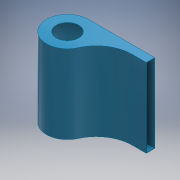
# Autodesk Inventor part: blower
Saved by Autodesk Inventor 2017 (Build 210142000, 142)
## iProperties
Created: 2017-04-22
Part Number: blower
Material: Generic
Document SubType Name: Modeling
Designer: master
Density: 1 g/cm^3
Appearance: Sky Blue Dark
Author: master
Autodesk Inventor part; units mm, degrees
ref_plane "YZ Plane" through (0, 0, 0) normal (1, 0, 0) x (0, 1, 0)
ref_plane "XZ Plane" through (0, 0, 0) normal (0, 1, 0) x (-1, 0, 0)
ref_plane "XY Plane" through (0, 0, 0) normal (0, 0, 1) x (1, 0, 0)
sketch "Sketch1" plane through (0, 0, 0) normal (0, 0, 1) x (1, 0, 0)
  arc A0 (0, 7.5) -> (6.8483, -3.0578) centre (0, 0) ccw
  line L0 (0, 7.5) -> (23.5, 7.5)
  line L1 (23.5, 7.5) -> (23.5, 4.5)
  line L2 (23.5, 4.5) -> (18.5, 4.5)
  arc A1 (18.5, 4.5) -> (6.8483, -3.0578) centre (18.5, -8.2604) ccw
  dimension "d0" = 15
  dimension "d3" = 3
  dimension "d5" = 23.5
  dimension "d12" = 5
  constraints: 6 end point, 4 point on circle, 3 tangent, 2 centre point, 1 coincident, 1 horizontal, 1 perpendicular, 1 vertical
  measures "d0" diameter of A0
  measures "d3" distance of L0.end L1.end
  measures "d5" distance from line of L1 point (0, 0)
  measures "d12" distance of L1.end L2.end
extrude "Extrusion1" add sketch "Sketch1" along normal blind 28
shell "Shell1" thickness 0.18 removed faces 1 at (23.5, 5.5, 18.6667)
sketch "Sketch2" plane through (0, 0, 28) normal (0, 0, 1) x (1, 0, 0)
  circle A0 centre (0, 0) radius 4
  dimension "d9" = 8
  constraints: 1 centre point, 1 coincident
  measures "d9" diameter of A0
extrude "Extrusion2" cut sketch "Sketch2" against normal blind 31
body "Solid1"
